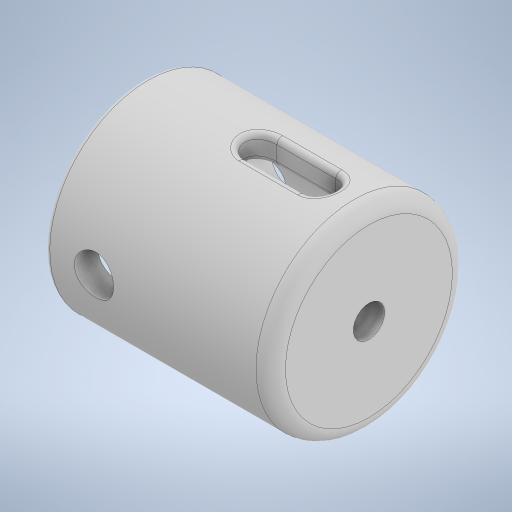
# Autodesk Inventor part: pressure_cyclinder_V1
Saved by Autodesk Inventor 2023 (Build 270158000, 158)
## iProperties
Created: 2023-05-10
Part Number: pressure_cyclinder_V1
Material: Generisch
Document SubType Name: Modeling
Designer: Mathi
Density: 1 g/cm^3
Appearance: Vorgabe
Author: Mathi
Autodesk Inventor part; units mm, degrees
ref_plane "YZ Plane" through (0, 0, 0) normal (1, 0, 0) x (0, 1, 0)
ref_plane "XZ Plane" through (0, 0, 0) normal (0, 1, 0) x (-1, 0, 0)
ref_plane "XY Plane" through (0, 0, 0) normal (0, 0, 1) x (1, 0, 0)
sketch "Skizze1" plane through (0, 0, 0) normal (0, 0, 1) x (1, 0, 0)
  line L0 (0, 0) -> (83.6234, 0)
  line L1 (-40, 15.1) -> (0, 15.1)
  line L2 (0, 15.1) -> (0, 0)
  line L3 (6, 0) -> (6, 20)
  line L4 (6, 20) -> (-40, 20)
  line L5 (-40, 20) -> (-40, 15.1)
  circle A0 centre (-30, 0) radius 4
  line L6 (-40, 19) -> (6, 19) construction
  dimension "d0" = 30.2
  dimension "d1" = 4.9
  dimension "d2" = 40
  dimension "d3" = 6
  dimension "d4" = 40
  dimension "d19" = 8
  dimension "d20" = 30
  dimension "d28" = 1
  constraints: 14 end point, 4 perpendicular, 3 point on line, 2 horizontal, 1 centre point, 1 horizontal alignment, 1 vertical
  measures "d0" diameter of L1 L0
  measures "d1" distance between parallel lines of L1 L4
  measures "d2" diameter of L4 L0
  measures "d3" distance between parallel lines of L3 L2
  measures "d4" distance between parallel lines of L2 L5
  measures "d19" diameter of A0
  measures "d20" distance from line of L2 A0.centre
  measures "d28" distance between parallel lines of L4 L6
revolve "Umdrehung1" add sketch "Skizze1" angle 360 about axis through (0, 0, 0) along (1, 0, 0) contours L2 L1 L5 L4 L3 L0
sketch "Skizze2" plane through (6, 0, 0) normal (1, 0, 0) x (0, 0, -1)
  point P0 (0, 0)
  point P1 (0, 0)
  constraints: 1 coincident
hole "Bohrung1" at (6, 0, 0) direction (-1, 0, 0) diameter 6.4 end through all
sketch "Skizze3" plane through (0, 0, 0) normal (0, 0, 1) x (1, 0, 0)
  circle A0 centre (-30, 0) radius 4 projected
  point P0 (0, 0)
extrude "Extrusion1" cut sketch "Skizze3" along normal through all both and the other way through all
sketch "Skizze4" plane through (0, 0, 0) normal (0, 1, 0) x (-1, 0, 0)
  line L0 (4, 0) -> (16, 0) construction
  line L1 (4, -3.25) -> (16, -3.25)
  line L2 (16, 3.25) -> (4, 3.25)
  arc A0 (4, 3.25) -> (4, -3.25) centre (4, 0) ccw
  arc A1 (16, -3.25) -> (16, 3.25) centre (16, 0) ccw
  point P0 (0, 0)
  point P1 (10, 0)
  dimension "d23" = 6.5
  dimension "d24" = 4
  dimension "d25" = 12
  constraints: 8 end point, 4 point on circle, 4 tangent, 2 centre point, 1 horizontal, 1 horizontal alignment, 1 midpoint, 1 parallel
  measures "d23" diameter of A1
  measures "d24" distance of L0.start point (0, 0)
  measures "d25" distance of L0.start L0.end
extrude "Extrusion2" cut sketch "Skizze4" along normal through all
fillet "Rundung1" radius 3 1 edges at (6, -20, 0)
fillet "Rundung2" radius 1 15 edges at (-40, -15.1, 0) (-40, -20, 0) (0, -15.1, 0) (-18.1126, 14.8967, -2.4697) (-18.1111, 14.8964, 2.471) (-10, 14.7461, 3.25) (-1.8964, 14.8954, 2.4774) (-1.8886, 14.8965, -2.4708) (-10, 14.7461, -3.25) (-1.8998, 19.8456, 2.4803) (-1.8904, 19.8466, -2.4723) (-10, 19.7342, 3.25) (-18.1098, 19.8466, 2.4721) (-18.1109, 19.8468, -2.4711) (-10, 19.7342, -3.25)
sketch "Skizze5" plane through (0, 0, 0) normal (0, 0, 1) x (1, 0, 0)
  line L0 (6, 19) -> (-40, 19)
  line L1 (-40, 19) -> (-40, 20)
  line L2 (-40, 20) -> (6, 20)
  line L3 (6, 20) -> (6, 19)
  line L4 (-40, 20) -> (-40, 15.1) projected
  line L5 (6, 20) -> (-40, 20) projected
  line L6 (6, 0) -> (6, 20) projected
  line L7 (-40, 19) -> (6, 19) construction
  point P0 (0, 0)
  constraints: 8 end point, 2 parallel, 1 horizontal, 1 perpendicular
sketch "Skizze6" plane through (-39.5, 19, 6.245) normal (0, 1, 0) x (1, 0, 0)
  point P0 (39.5, 6.245)
  point P1 (17.5, 6.245)
  point P2 (11.5, 6.245)
  dimension "d31" = 22
  dimension "d32" = 6
  constraints: 2 horizontal alignment
  measures "d31" distance of point (17.5, 6.245) point (39.5, 6.245)
  measures "d32" distance of point (11.5, 6.245) point (17.5, 6.245)
